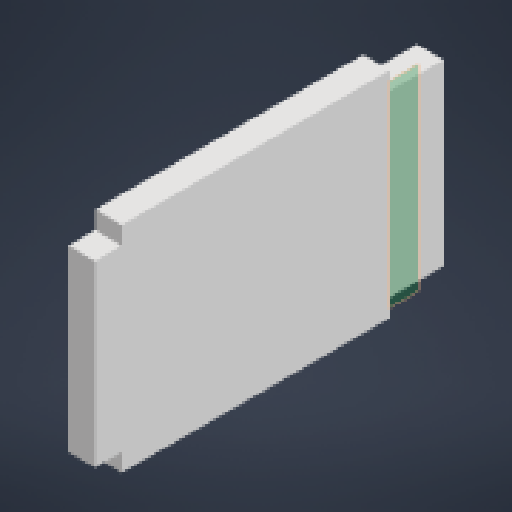
# Autodesk Inventor part: thanhnang
Saved by Autodesk Inventor 2023 (Build 270158000, 158)
## iProperties
Created: 2023-09-09
Part Number: thanhnang
Material: Generic
Document SubType Name: Modeling
Designer: philo
Density: 1 g/cm^3
Appearance: Default
Author: philo
Autodesk Inventor part; units mm, degrees
ref_plane "YZ Plane" through (0, 0, 0) normal (1, 0, 0) x (0, 1, 0)
ref_plane "XZ Plane" through (0, 0, 0) normal (0, 1, 0) x (-1, 0, 0)
ref_plane "XY Plane" through (0, 0, 0) normal (0, 0, 1) x (1, 0, 0)
ref_plane "Work Plane1" through (-17, -57.5, 0) normal (-1, 0, 0) x (0, -1, 0)
sketch "Sketch2" plane through (-17, -57.5, 0) normal (-1, 0, 0) x (0, -1, 0)
  line L0 (0, -3) -> (0, -6) projected
  line L1 (20, -3) -> (20, -6) projected
  line L2 (20, 33) -> (20, 30) projected
  line L3 (0, 33) -> (0, 30) projected
  line L4 (0, 0) -> (0, -3) projected
  line L5 (20, 0) -> (20, -3) projected
  line L6 (0, -6) -> (20, -6)
  line L7 (20, -6) -> (20, 33)
  line L8 (20, 33) -> (0, 33)
  line L9 (0, 33) -> (0, -6)
  line L10 (-2, 0) -> (22, 0)
  line L11 (22, 0) -> (22, 30)
  line L12 (22, 30) -> (-2, 30)
  line L13 (-2, 30) -> (-2, 0)
  point P0 (-57.5, 0)
  point P1 (0, 30)
  point P2 (20, -6)
  point P3 (20, 0)
  point P4 (20, 30)
  point P5 (0, 33)
  dimension "d0" = 24
  dimension "d1" = 2
  constraints: 16 end point, 4 parallel, 2 horizontal, 2 perpendicular
  measures "d0" distance of L12.end L11.end
  measures "d1" distance between parallel lines of L13 L9
extrude "Extrusion1" add sketch "Sketch2" along normal blind 3
body "Solid1"
